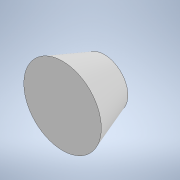
# Autodesk Inventor part: extruderHead
Saved by Autodesk Inventor 2020 (Build 240168000, 168)
## iProperties
Created: 2020-02-25
Part Number: extruderHead
Material: Generic
Document SubType Name: Modeling
Designer: zhang
Density: 1 g/cm^3
Appearance: Default
Author: zhang
Autodesk Inventor part; units mm, degrees
ref_plane "YZ Plane" through (0, 0, 0) normal (1, 0, 0) x (0, 1, 0)
ref_plane "XZ Plane" through (0, 0, 0) normal (0, 1, 0) x (-1, 0, 0)
ref_plane "XY Plane" through (0, 0, 0) normal (0, 0, 1) x (1, 0, 0)
sketch "Sketch2" plane through (0, 0, 0) normal (0, 1, 0) x (-1, 0, 0)
  line L0 (0, 0) -> (0, 21)
  line L1 (0, 21) -> (-14.8235, 21)
  line L2 (-14.8235, 21) -> (-9, 5)
  line L3 (-9, 5) -> (-4, 5)
  line L4 (-4, 5) -> (-4, 2)
  line L5 (-4, 2) -> (-1.4004, 2)
  line L6 (-1.4004, 2) -> (0, 0)
  dimension "d21" = 21
  dimension "d22" = 2
  dimension "d23" = 3
  dimension "d24" = 4
  dimension "d25" = 70
  dimension "d28" = 9
  dimension "d30" = 125
  constraints: 14 end point, 3 perpendicular, 1 parallel, 1 vertical
  measures "d21" distance of L0.start L0.end
  measures "d22" vertical distance of L5.end L0.start
  measures "d23" distance of L3.end L4.end
  measures "d24" distance between parallel lines of L0 L4
  measures "d25" angle of L1 L2
  measures "d28" distance from line of L0 L2.end
  measures "d30" angle of L5 L6
revolve "Revolution2" add sketch "Sketch2" angle 360 about axis through (0, 0, 0) along (0, 0, 1)
body "Solid2"
